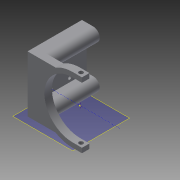
# Autodesk Inventor part: base
Saved by Autodesk Inventor 2015 SP2 (Build 190223200, 223)
## iProperties
Created: 2016-03-05
Part Number: base
Material: Generic
Document SubType Name: Modeling
Designer: marc
Density: 1 g/cm^3
Appearance: Default
Author: marc
Autodesk Inventor part; units mm, degrees
ref_plane "YZ Plane" through (0, 0, 0) normal (1, 0, 0) x (0, 1, 0)
ref_plane "XZ Plane" through (0, 0, 0) normal (0, 1, 0) x (-1, 0, 0)
ref_plane "XY Plane" through (0, 0, 0) normal (0, 0, 1) x (1, 0, 0)
sketch "Sketch1" plane through (0, 0, 0) normal (0, 1, 0) x (-1, 0, 0)
  arc A0 (0, -30) -> (0, 30) centre (0, 0) ccw
  arc A1 (0, -35) -> (0, 35) centre (0, 0) ccw
  line L0 (0, 66.4807) -> (0, -80.0863) construction
  line L1 (-55.1659, 0) -> (60.8047, 0) construction
  line L2 (18.0278, 30) -> (48.0278, 30)
  line L3 (48.0278, 30) -> (48.0278, -30)
  line L4 (48.0278, -30) -> (18.0278, -30)
  line L5 (18.0278, 30) -> (48.0278, -30) construction
  line L6 (48.0278, 30) -> (18.0278, -30) construction
  line L7 (18.0278, 30) -> (18.0278, -30) construction
  line L8 (0, 35) -> (-10, 35)
  line L9 (0, 30) -> (-10, 30)
  line L10 (-10, 35) -> (-10, 30)
  line L11 (0, -35) -> (-10, -35)
  line L12 (0, -30) -> (-10, -30)
  line L13 (-10, -35) -> (-10, -30)
  point P0 (33.0278, 0)
  dimension "diameterCylinder" = 60
  dimension "thicknessFlange" = 5
  dimension "widthC" = 60
  dimension "offsetC" = 30
  dimension "d33" = 10
  constraints: 28 end point, 7 point on line, 6 point on circle, 4 horizontal, 2 centre point, 2 coincident, 2 midpoint, 2 parallel, 2 symmetric about line, 2 vertical, 1 perpendicular
  measures "diameterCylinder" diameter of A0
  measures "thicknessFlange" radial gap between concentric circles of A1 A0
  measures "widthC" distance of L2.end L3.end
  measures "offsetC" distance from line of L4.end L3
  measures "d33" distance between parallel lines of L0 L10
extrude "Extrusion1" add sketch "Sketch1" along normal blind 8
sketch "Sketch2" plane through (0, 8, 0) normal (0, 1, 0) x (1, 0, 0)
  line L0 (-18.0278, 30) -> (-48.0278, 30) projected
  line L1 (-48.0278, -30) -> (-43.0278, -30)
  line L2 (-43.0278, -30) -> (-43.0278, 30)
  line L3 (-43.0278, 30) -> (-48.0278, 30)
  line L4 (-48.0278, 30) -> (-48.0278, -30)
  point P0 (0, 0)
  dimension "thicknessC" = 5
  constraints: 8 end point, 2 parallel, 1 horizontal, 1 perpendicular, 1 point on line
  measures "thicknessC" distance between parallel lines of L4 L2
extrude "Extrusion2" add sketch "Sketch2" along normal blind 50
sketch "Sketch3" plane through (0, 8, 0) normal (0, 1, 0) x (1, 0, 0)
  circle A0 centre (-36.0278, -23) radius 4
  circle A1 centre (-36.0278, -23) radius 7
  line L0 (-36.0278, -30) -> (-48.0278, -30)
  line L1 (-48.0278, 30) -> (-48.0278, -30) projected
  line L2 (-48.0278, -30) -> (-48.0278, -16)
  line L3 (-48.0278, -16) -> (-36.0278, -16)
  line L4 (0, 0) -> (-116.9201, 0) construction
  line L5 (-43.0278, -30) -> (-43.0278, 30) construction
  line L6 (-43.0278, -30) -> (-18.0278, -30) construction
  circle A2 centre (-36.0278, 23) radius 4
  circle A3 centre (-36.0278, 23) radius 7
  line L7 (-36.0278, 30) -> (-48.0278, 30)
  line L8 (-48.0278, -30) -> (-48.0278, 30)
  line L9 (-48.0278, 16) -> (-36.0278, 16)
  dimension "tRodHolder" = 3
  dimension "DRodHolder" = 8
  constraints: 14 end point, 8 symmetric about line, 4 centre point, 4 point on circle, 4 point on line, 3 tangent, 2 coincident, 2 horizontal, 1 collinear, 1 parallel, 2 other
  measures "tRodHolder" radial gap between concentric circles of A1 A0
  measures "DRodHolder" diameter of A0
extrude "Extrusion3" add sketch "Sketch3" along normal up to surface (50 mm away)
sketch "Sketch4" plane through (-48.0278, 0, -30) normal (-1, 0, 0) x (0, 0, 1)
  line L0 (30, 0) -> (30, 84.984) construction
  line L1 (18, 20) -> (42, 20) construction
  line L2 (42, 20) -> (42, 40) construction
  line L3 (42, 40) -> (18, 40) construction
  line L4 (18, 40) -> (18, 20) construction
  line L5 (18, 20) -> (42, 40) construction
  line L6 (42, 20) -> (18, 40) construction
  line L7 (0, 0) -> (60, 0) construction
  point P0 (30, 30)
  dimension "holespacingZ" = 24
  dimension "holeSpacingY" = 20
  dimension "holeOffset" = 30
  constraints: 14 end point, 4 coincident, 2 midpoint, 2 parallel, 1 horizontal, 1 perpendicular, 1 point on line, 1 vertical
  measures "holespacingZ" distance of L2.end L3.end
  measures "holeSpacingY" distance between parallel lines of L1 L3
  measures "holeOffset" distance from line of L7 point (30, 30)
hole "Hole1" at (-48.0278, 40, -12) at (-48.0278, 40, 12) at (-48.0278, 20, 12) at (-48.0278, 20, -12) direction (1, 0, 0) diameter 3.4 end through all clearance for "Socket Head Cap Screw ISO 4762" size "M3" standard "ISO"
ref_plane "Work Plane1" through (0, 0, -35) normal (0, 0, -1) x (-1, 0, 0)
sketch "Sketch5" plane through (0, 0, -35) normal (0, 0, -1) x (-1, 0, 0)
  line L0 (0, 0) -> (0, 8) projected
  line L1 (-10, 0) -> (-10, 8) projected
  point P0 (-5, 4)
  dimension "holePosistionYF" = 4
  dimension "d34" = 5
  measures "holePosistionYF" vertical distance of L0.start point (-5, 4)
  measures "d34" distance from line of L1 point (-5, 4)
hole "Hole2" at (5, 4, -35) direction (0, 0, 1) diameter 4.5 end through all clearance for "Socket Head Cap Screw ISO 4762" size "M4" standard "ISO"
sketch "Sketch7" plane through (0, 8, 0) normal (0, 1, 0) x (1, 0, 0)
  line L0 (-50.9329, 0) -> (42.7836, 0) construction
  point P0 (0, 0)
  point P1 (0, 0)
  constraints: 2 end point, 1 coincident, 1 horizontal, 1 point on line
equation "\"holePosistionYF\" = 0.5 * flangeHeigth"
equation "\"flangeHeigth\" = 8"
body "Solid1"
